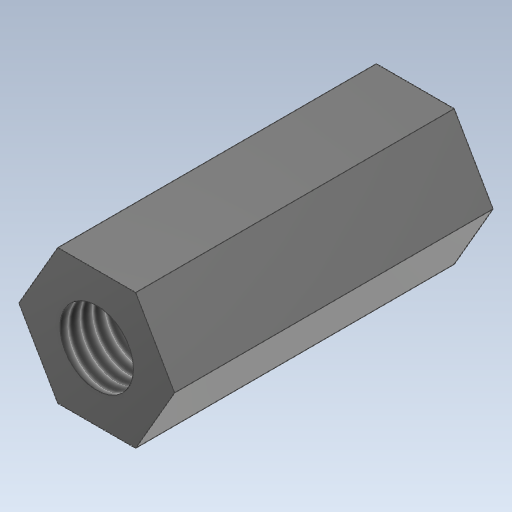
# Autodesk Inventor part: ASL-313BE
Saved by Autodesk Inventor 2020.4 (Build 244396000, 396)
## iProperties
Created: 2022-01-04
Part Number: ASL-313BE
Material: アルミニウム
Document SubType Name: Modeling
Designer: Masato Kubotera
Density: 2.7 g/cm^3
Appearance: 滑らか - 黒
Description: 既製品
Catalog Web Link: https://www.hirosugi-net.co.jp/shop/g/g13223/
Mass: 0.671417 g
Surface Area: 4.08463 cm^2
Volume: 0.248673 cm^3
Author: Masato Kubotera
Autodesk Inventor part; units mm, degrees
ref_plane "YZ Plane" through (0, 0, 0) normal (1, 0, 0) x (0, 1, 0)
ref_plane "XZ Plane" through (0, 0, 0) normal (0, 1, 0) x (-1, 0, 0)
ref_plane "XY Plane" through (0, 0, 0) normal (0, 0, 1) x (1, 0, 0)
sketch "スケッチ1" plane through (0, 0, 0) normal (0, 0, 1) x (1, 0, 0)
  line L0 (-3.1754, 0) -> (-1.5877, 2.75)
  line L1 (-1.5877, 2.75) -> (1.5877, 2.75)
  line L2 (1.5877, 2.75) -> (3.1754, 0)
  line L3 (3.1754, 0) -> (1.5877, -2.75)
  line L4 (1.5877, -2.75) -> (-1.5877, -2.75)
  line L5 (-1.5877, -2.75) -> (-3.1754, 0)
  circle A0 centre (0, 0) radius 1.5
  dimension "d0" = 5.5
  dimension "d1" = 3
  constraints: 12 end point, 2 coincident, 1 centre point, 1 horizontal, 13 other
  measures "d0" distance between parallel lines of L2 L5
  measures "d1" diameter of A0
extrude "押し出し1" add sketch "スケッチ1" along normal blind 13
thread "ねじ1" size "M3x0.5" class "6H" standard "ANSI Metric M Profile" full length
